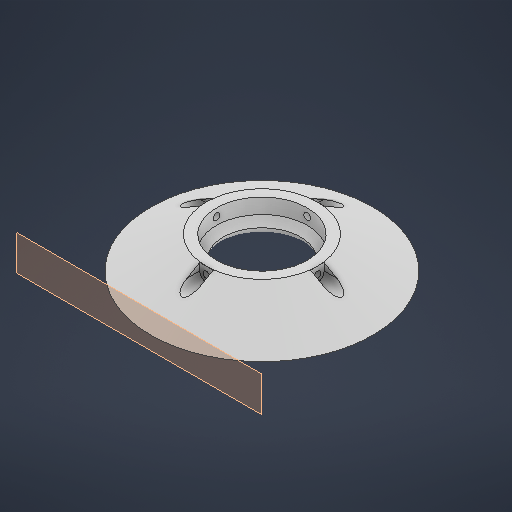
# Autodesk Inventor part: Статор без зубьев
Saved by Autodesk Inventor 2026 (Build 300175000, 175)
## iProperties
Created: 2025-08-22
Part Number: Статор без зубьев
Material: Типовые
Document SubType Name: Modeling
Designer: kvm13
Density: 1 g/cm^3
Appearance: По умолчанию
Author: kvm13
Autodesk Inventor part; units mm, degrees
ref_plane "YZ Plane" through (0, 0, 0) normal (1, 0, 0) x (0, 1, 0)
ref_plane "XZ Plane" through (0, 0, 0) normal (0, 1, 0) x (-1, 0, 0)
sketch "Эскиз1" plane through (0, 0, 0) normal (1, 0, 0) x (0, 1, 0)
  line L0 (0, 0) -> (0, 11.5)
  line L1 (0, 11.5) -> (0, 13.5)
  line L2 (0, 13.5) -> (2, 13.5)
  line L3 (2, 13.5) -> (0, 11.5)
  line L4 (2, 13.5) -> (6.5, 13.5)
  line L5 (6.5, 13.5) -> (6.5, 16.5)
  line L6 (6.5, 16.5) -> (2, 16.5)
  line L7 (0, 13.5) -> (0, 16.5)
  line L8 (0, 16.5) -> (2, 16.5)
  line L9 (0, 27.7583) -> (0, 33)
  line L10 (6.5, 16.5) -> (-3.0263, 33)
  line L11 (6.5, 16.5) -> (32.9156, 16.5) construction
  line L12 (0, 33) -> (-3.0263, 33)
  line L13 (-3.0263, 33) -> (-3.0263, 16.5)
  line L14 (-3.0263, 16.5) -> (-2.9965, 14.7974) construction
  line L15 (-2.9965, 14.7974) -> (-2.6552, 12.8623) construction
  line L16 (-2.6552, 12.8623) -> (-1.03, 11.5) construction
  line L17 (-1.03, 11.5) -> (0, 11.5) construction
  spline S0 degree 4 poles (-3.0263, 16.5) (-2.9965, 14.7974) (-2.6552, 12.8623) (-1.03, 11.5) (0, 11.5) knots 1 1 1 1 1 2 2 2 2 2
  line L18 (0, 0) -> (14.3588, 0)
  dimension "d1" = 2
  dimension "d2" = 2
  dimension "d3" = 13.5
  dimension "d4" = 3
  dimension "d5" = 4.5
  dimension "d6" = 16.5
  dimension "d7" = 120
  constraints: 30 end point, 5 perpendicular, 5 point on line, 3 horizontal, 2 vertical, 3 other
  measures "d1" distance of L0.end L1.end
  measures "d2" distance of L1.end L2.end
  measures "d3" distance of L0.start L1.end
  measures "d4" distance of L2.end L6.end
  measures "d5" distance of L2.end L4.end
  measures "d6" distance of L7.end L9.end
  measures "d7" angle of L11 L10
revolve "Вращение1" add sketch "Эскиз1" angle 360 about axis through (0, 0, 0) along (0, 1, 0) contours S0 L13 L10 L6 L8 L7 L1 | L1 L2 L3 | L7 L8 L6 L5 L4 L2
sketch "Эскиз2" plane through (0, 0, 0) normal (0, 0, 1) x (1, 0, 0)
  line L0 (13.5, 6.5) -> (-13.5, 6.5) projected
  line L1 (13.5, 2) -> (-13.5, 2) projected
  line L2 (0, 2) -> (0, 6.5)
  circle A0 centre (0, 4.25) radius 1
  point P0 (0, 0)
  dimension "d9" = 2
  constraints: 3 midpoint, 2 end point, 1 centre point
  measures "d9" diameter of A0
extrude "Выдавливание1" cut sketch "Эскиз2" along normal blind 30
ref_plane "РабПлоскость1" through (0, 0, 36.5125) normal (0, 0, 1) x (1, 0, 0)
sketch "Эскиз3" plane through (0, 0, 36.5125) normal (0, 0, 1) x (1, 0, 0)
  line L0 (16.5, 6.5) -> (-16.5, 6.5) projected
  arc A0 (-2, 4.25) -> (2, 4.25) centre (0, 4.25) ccw
  line L1 (-2, 4.25) -> (-2, 6.5)
  line L2 (2, 4.25) -> (2, 6.5)
  point P0 (0, 0)
  dimension "d14" = 4
  constraints: 4 end point, 2 perpendicular, 2 point on circle, 2 point on line, 2 tangent, 1 centre point, 1 other
  measures "d14" diameter of A0
extrude "Выдавливание2" cut sketch "Эскиз3" against normal blind 20.013
pattern_circular "Круговой массив1" count 4 over 360 about axis through (0, 4.25, 0) along (0, 1, 0) of "Выдавливание2", "Выдавливание1"
